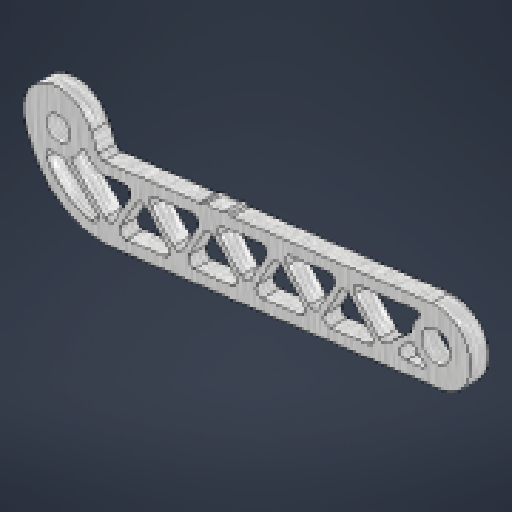
# Autodesk Inventor part: PLATE,LINK,REAR,INTAKE
Saved by Autodesk Inventor 2026 (Build 300175000, 175)
## iProperties
Created: 2026-02-15
Part Number: PLATE,LINK,REAR,INTAKE
Material: Aluminum 7075
Document SubType Name: Modeling
Designer: Jthib
Mass: 142.593 g
Surface Area: 245.092 cm^2
Volume: 50.7448 cm^3
Density: 2.81 g/cm^3
Appearance: Satin - Brushed Heavy
Author: Jthib
Autodesk Inventor part; units mm, degrees
ref_plane "YZ Plane" through (0, 0, 0) normal (1, 0, 0) x (0, 1, 0)
ref_plane "XZ Plane" through (0, 0, 0) normal (0, 1, 0) x (-1, 0, 0)
ref_plane "XY Plane" through (0, 0, 0) normal (0, 0, 1) x (1, 0, 0)
sketch "Sketch1" plane through (0, 0, 0) normal (0, 0, 1) x (1, 0, 0)
  line L0 (-101.6, 0) -> (101.6, 0) construction
  arc A0 (-83.9597, 7.1919) -> (-119.2403, -7.1919) centre (-101.6, 0) ccw
  line L1 (-101.6, 0) -> (-98.1108, -8.5582) construction
  arc A1 (-98.1108, -8.5582) -> (-74.7524, -22.2183) centre (-77.5305, -0.1676) ccw construction
  line L2 (-74.7524, -22.2183) -> (101.6, 0) construction
  line L3 (-80.4706, -1.3663) -> (-83.9597, 7.1919)
  line L4 (-119.2403, -7.1919) -> (-115.7511, -15.7502)
  arc A2 (-115.7511, -15.7502) -> (-72.3711, -41.1189) centre (-77.5305, -0.1676) ccw
  line L5 (-72.3711, -41.1189) -> (103.9813, -18.9006)
  arc A3 (103.9813, -18.9006) -> (99.2188, 18.9006) centre (101.6, 0) ccw
  arc A4 (-80.4706, -1.3663) -> (-77.1336, -3.3177) centre (-77.5305, -0.1676) ccw
  line L6 (-95.25, 3.6662) -> (-95.25, -3.6662)
  line L7 (-95.25, -3.6662) -> (-101.6, -7.3323)
  line L8 (-101.6, -7.3323) -> (-107.95, -3.6662)
  line L9 (-107.95, -3.6662) -> (-107.95, 3.6662)
  line L10 (-107.95, 3.6662) -> (-101.6, 7.3323)
  line L11 (-101.6, 7.3323) -> (-95.25, 3.6662)
  line L12 (-101.6, 0) -> (-19.155, 23.4862) construction
  line L13 (99.2188, 18.9006) -> (-11.8775, 4.9038)
  line L14 (-11.8775, 4.9038) -> (-77.1336, -3.3177)
  circle A5 centre (-19.155, 23.4862) radius 19.05
  line L15 (-23.2102, 4.8728) -> (-24.412, 3.3246)
  line L16 (-10.6098, 6.4603) -> (-9.0615, 5.2586)
  line L17 (-19.155, 23.4862) -> (-16.7367, 4.2916) construction
  point P0 (0, 0)
  dimension "d1" = 38.1
  dimension "d2" = 203.2
  dimension "d14" = 22.225
  dimension "d15" = 105
  dimension "d16" = 25.4
  dimension "d18" = 12.7
  dimension "d37" = 85.725
  dimension "d40" = 3.175
  dimension "d42" = 8.72
  dimension "d46" = 38.1
  dimension "d47" = 90
  dimension "d48" = 12.7
  constraints: 39 end point, 12 point on circle, 10 tangent, 6 centre point, 3 point on line, 2 coincident, 2 perpendicular, 1 concentric, 1 horizontal, 1 midpoint, 16 other
  measures "d1" diameter of A0
  measures "d2" distance of L0.start L0.end
  measures "d14" radius of A1
  measures "d15" angle of L2 L1
  measures "d16" distance from line of L0.start L2
  measures "d18" distance between parallel lines of L9 L6
  measures "d37" distance of L12.start L12.end
  measures "d40" radius of A4
  measures "d42" angle of L14 L12
  measures "d46" diameter of A5
  measures "d47" angle of L16 L15
  measures "d48" distance of L16.start L15.start
extrude "Extrusion1" add sketch "Sketch1" along normal mid plane 9.525 contours L3 A4 L14 L13 A3 L5 A2 L4 A0 | L15 A5 L16 L13 L14 | L6 L7 L8 L9 L10 L11
sketch "Sketch2" plane through (0, 0, 4.7625) normal (0, 0, 1) x (1, 0, 0)
  arc A0 (-83.9597, 7.1919) -> (-119.2403, -7.1919) centre (-101.6, 0) ccw construction
  arc A1 (103.9813, -18.9006) -> (99.2188, 18.9006) centre (101.6, 0) ccw construction
  point P0 (0, 0)
  constraints: 2 coincident
hole "Hole1" at (-101.6, 0, 4.7625) direction (0, 0, -1) diameter 12.7 end through all start extended yes
hole "Hole2" at (101.6, 0, 4.7625) direction (0, 0, -1) diameter 15.875 end through all start extended yes
sketch "Sketch3" plane through (0, 0, -4.7625) normal (0, 0, -1) x (-1, 0, 0)
  line L0 (77.1336, -3.3177) -> (-99.2188, 18.9006) construction
  arc A0 (77.1336, -3.3177) -> (80.4706, -1.3663) centre (77.5305, -0.1676) ccw construction
  line L1 (83.9597, 7.1919) -> (80.4706, -1.3663) construction
  arc A1 (119.2403, -7.1919) -> (83.9597, 7.1919) centre (101.6, 0) ccw construction
  line L2 (115.7511, -15.7502) -> (119.2403, -7.1919) construction
  arc A2 (72.3711, -41.1189) -> (115.7511, -15.7502) centre (77.5305, -0.1676) ccw construction
  line L3 (-103.9813, -18.9006) -> (72.3711, -41.1189) construction
  arc A3 (-99.2188, 18.9006) -> (-103.9813, -18.9006) centre (-101.6, 0) ccw construction
  line L4 (-100.0125, 12.6004) -> (76.3399, -9.6179)
  arc A4 (76.3399, -9.6179) -> (86.3506, -3.7636) centre (77.5305, -0.1676) ccw
  line L5 (86.3506, -3.7636) -> (89.8398, 4.7946)
  circle A5 centre (101.6, 0) radius 12.7
  line L6 (113.3602, -4.7946) -> (109.871, -13.3529)
  arc A6 (73.1649, -34.8187) -> (109.871, -13.3529) centre (77.5305, -0.1676) ccw
  line L7 (73.1649, -34.8187) -> (-103.1875, -12.6004)
  circle A7 centre (-101.6, 0) radius 12.7
  point P0 (0, 0)
  dimension "d19" = 6.35
  constraints: 8 end point, 8 point on circle, 4 centre point, 3 tangent, 4 other
  measures "d19" distance between parallel lines of L3 L7
extrude "Extrusion2" cut sketch "Sketch3" against normal blind 9.525 contours L4 A4 L5 A5 L6 A6 L7 A7
sketch "Sketch4" plane through (0, 0, -4.7625) normal (0, 0, -1) x (-1, 0, 0)
  arc A0 (89.8398, 4.7946) -> (113.3602, -4.7946) centre (101.6, 0) ccw construction
  line L0 (73.1649, -34.8187) -> (-103.1875, -12.6004) construction
  arc A1 (73.1649, -34.8187) -> (109.871, -13.3529) centre (77.5305, -0.1676) ccw construction
  arc A2 (76.3399, -9.6179) -> (86.3506, -3.7636) centre (77.5305, -0.1676) ccw construction
  line L1 (-100.0125, 12.6004) -> (76.3399, -9.6179) construction
  arc A3 (-103.1875, -12.6004) -> (-100.0125, 12.6004) centre (-101.6, 0) ccw construction
  line L2 (96.8054, -11.7602) -> (73.1649, -34.8187)
  line L3 (73.1649, -34.8187) -> (58.0399, -7.3123)
  line L4 (58.0399, -7.3123) -> (36.5649, -30.2075)
  line L5 (36.5649, -30.2075) -> (21.4398, -2.7012)
  line L6 (21.4398, -2.7012) -> (-0.0352, -25.5964)
  line L7 (-0.0352, -25.5964) -> (-15.1602, 1.91)
  line L8 (-15.1602, 1.91) -> (-36.6352, -20.9852)
  line L9 (-36.6352, -20.9852) -> (-51.7602, 6.5212)
  line L10 (-73.2352, -16.374) -> (-51.7602, 6.5212)
  line L11 (-73.2352, -16.374) -> (-88.9996, -1.5875)
  point P0 (0, 0)
  constraints: 20 end point, 8 point on line, 5 equal length, 3 parallel, 3 point on circle, 1 perpendicular
ref_plane "Work Plane1" through (-96.8054, -11.7602, -4.7625) normal (0.715863, -0.6982408, 0) x (0.6982408, 0.715863, 0)
sketch "Sketch5" plane through (-96.8054, -11.7602, -4.7625) normal (0.715863, -0.6982408, 0) x (0.6982408, 0.715863, 0)
  line L0 (-1.5875, 9.525) -> (1.5875, 9.525)
  line L1 (1.5875, 9.525) -> (1.5875, 0)
  line L2 (1.5875, 0) -> (-1.5875, 0)
  line L3 (-1.5875, 0) -> (-1.5875, 9.525)
  point P0 (76.0121, 4.7625)
  point P1 (0, 0)
  point P2 (0, 0)
  point P3 (0, 0)
  point P4 (0, 0)
  dimension "d24" = 9.525
  dimension "d25" = 3.175
  constraints: 8 end point, 2 parallel, 1 coincident, 1 horizontal, 1 midpoint, 1 perpendicular
  measures "d24" distance of L2.end L0.start
  measures "d25" distance of L0.start L0.end
sweep "Sweep1" add profiles "Sketch5" path "Sketch4"
delete faces "Delete Face1" heal yes whole lump no faces at (-97.5443, -12.5178, 1.5875) (88.2756, -0.8156, -1.5875)
fillet "Fillet1" radius 3.175 34 edges at (-98.5073, -12.3177, 0) (-75.235, -35.0171, 0) (-73.5504, -32.2251, 0) (-71.2184, -34.5735, 0) (-113.3602, -4.7946, 0) (-59.9864, -7.5576, 0) (-57.7022, -9.9929, 0) (-56.0933, -7.0671, 0) (-38.5114, -30.4528, 0) (-34.6183, -29.9623, 0) (-36.9026, -27.527, 0) (-1.9113, -25.8416, 0) (-0.3025, -22.9158, 0) (1.9817, -25.3511, 0) (15.4979, -0.7705, 0) (34.6887, -21.2304, 0) (38.5817, -20.74, 0) (36.2975, -18.3047, 0) (49.8137, 6.2759, 0) (52.0979, 3.8406, 0) (53.7067, 6.7664, 0) (71.2887, -16.6193, 0) (75.9158, -16.0363, 0) (73.307, -14.1301, 0) (88.91, 0.505, 0) (-21.1021, -5.3817, 0) (-23.3864, -2.9464, 0) (13.2137, 1.6648, 0) (17.1067, 2.1552, 0) (-19.4933, -2.4559, 0) (-24.412, 3.3246, 0) (-23.2102, 4.8728, 0) (-9.0615, 5.2586, 0) (-10.6098, 6.4603, 0)
fillet "Fillet1" radius 1.5875 4 edges at (-89.8398, 4.7946, 0) (100.0125, 12.6004, 0) (103.1875, -12.6004, 0) (89.3686, -3.418, 0)
body "Solid1"
